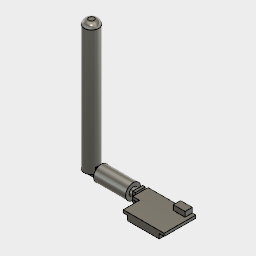
Video TX Module v1 (Autodesk Fusion 360 design; units mm, degrees)
Autodesk Fusion 360 part; units mm, degrees
note: some values were not read from the file. Set by a fixed rule: which sketch regions a step uses.
sketch "Sketch1" plane through (0, 0, 0) normal (0, 1, 0) x (1, 0, 0)
  line L0 (13.25, -10.25) -> (-13.25, -10.25)
  line L1 (-13.25, -10.25) -> (-13.25, 10.25)
  line L2 (-13.25, 10.25) -> (13.25, 10.25)
  line L3 (13.25, 10.25) -> (13.25, -10.25)
  line L4 (13.25, -10.25) -> (-13.25, 10.25) construction
  line L5 (-13.25, -10.25) -> (13.25, 10.25) construction
  line L6 (-13.25, 10.25) -> (-17.65, 10.25)
  line L7 (-17.65, 10.25) -> (-17.65, 0.25)
  line L8 (-17.65, 0.25) -> (-13.25, 0.25)
  dimension "d1" = 26.5
  dimension "d2" = 20.5
  dimension "d3" = 10
  dimension "d4" = 4.4
  measures "d1" distance of L1.end L2.end
  measures "d2" distance of L0.end L1.end
  measures "d3" distance of L6.end L7.end
  measures "d4" distance of L1.end L6.end
extrude "Extrude1" add sketch "Sketch1" along normal blind 1.85
sketch "Sketch2" plane through (0, 1.85, 0) normal (0, 1, 0) x (-1, 0, 0)
  line L0 (-13.25, -10.25) -> (17.65, -10.25)
  line L1 (17.65, -10.25) -> (17.65, -0.25)
  line L2 (17.65, -0.25) -> (13.25, -0.25)
  line L3 (13.25, -0.25) -> (13.25, 10.25)
  line L4 (13.25, 10.25) -> (-13.25, 10.25)
  line L5 (-13.25, 10.25) -> (-13.25, -10.25)
  line L6 (-11, -10.25) -> (-3.4, -10.25)
  line L7 (-3.4, -10.25) -> (-3.4, -5.55)
  line L8 (-3.4, -5.55) -> (-11, -5.55)
  line L9 (-11, -5.55) -> (-11, -10.25)
  dimension "d7" = 7.6
  dimension "d8" = 4.7
  dimension "d9" = 2.25
  measures "d7" distance of L6.start L6.end
  measures "d8" distance of L6.start L8.end
  measures "d9" distance of L5 L9
extrude "Extrude2" add sketch "Sketch2" along normal blind 3.2 contours L0 L6 L7 L8 L9
sketch "Sketch3" plane through (0, 0, 0) normal (0, -1, 0) x (1, 0, 0)
  line L0 (-17.65, -10.25) -> (13.25, -10.25)
  line L1 (13.25, -10.25) -> (13.25, 10.25)
  line L2 (13.25, 10.25) -> (-13.25, 10.25)
  line L3 (-13.25, 10.25) -> (-13.25, -0.25)
  line L4 (-13.25, -0.25) -> (-17.65, -0.25)
  line L5 (-17.65, -0.25) -> (-17.65, -10.25)
  line L6 (-10.5, 10.25) -> (10, 10.25)
  line L7 (10, 10.25) -> (10, -10.25)
  line L8 (10, -10.25) -> (-10.5, -10.25)
  line L9 (-10.5, -10.25) -> (-10.5, 10.25)
  dimension "d12" = 20.5
  dimension "d13" = 3.25
  measures "d12" distance of L7 L9
  measures "d13" distance of L1 L7
extrude "Extrude3" add sketch "Sketch3" along normal blind 3 contours L0 L2 L6 L7 L8 L9
sketch "Sketch4" plane through (-17.65, 0, 0) normal (-1, 0, 0) x (0, 0, 1)
  line L0 (-10.25, 0) -> (-0.25, 0)
  line L1 (-0.25, 0) -> (-0.25, 1.85)
  line L2 (-0.25, 1.85) -> (-10.25, 1.85)
  line L3 (-10.25, 1.85) -> (-10.25, 0)
  line L4 (-8.5, 3.05) -> (-2, 3.05)
  line L5 (-2, 3.05) -> (-2, -3.45)
  line L6 (-2, -3.45) -> (-8.5, -3.45)
  line L7 (-8.5, -3.45) -> (-8.5, 3.05)
  dimension "d16" = 6.5
  dimension "d17" = 6.5
  dimension "d18" = 1.2
  dimension "d19" = 1.75
  measures "d16" distance of L4.start L4.end
  measures "d17" distance of L4.start L6.end
  measures "d18" distance of L2 L4
  measures "d19" distance of L3 L7
extrude "Extrude4" add sketch "Sketch4" along normal blind 1.7 contours L0 L2 L5 L7 | L0 L5 L6 L7 | L2 L4 L5 L7
sketch "Sketch5" plane through (-19.35, 0, 0) normal (-1, 0, 0) x (0, 0, 1)
  line L0 (-8.5, -3.45) -> (-2, -3.45)
  line L1 (-2, -3.45) -> (-2, 3.05)
  line L2 (-2, 3.05) -> (-8.5, 3.05)
  line L3 (-8.5, 3.05) -> (-8.5, -3.45)
  circle A0 centre (-5.25, -0.2) radius 2.65
  line L4 (-5.25, -0.2) -> (-5.25, 3.05) construction
  line L5 (-5.25, -0.2) -> (-5.25, -3.45) construction
  dimension "d22" = 5.3
  measures "d22" diameter of A0
extrude "Extrude5" add sketch "Sketch5" along normal blind 2.85 contours A0
sketch "Sketch6" plane through (-22.2, 0, 0) normal (-1, 0, 0) x (0, 0, 1)
  circle A0 centre (-5.25, -0.2) radius 2.65
  circle A1 centre (-5.25, -0.2) radius 5
  dimension "d25" = 10
  measures "d25" diameter of A1
extrude "Extrude6" add sketch "Sketch6" along normal blind 20.75 contours A0 | A1
sketch "Sketch7" plane through (-42.95, 0, 0) normal (-1, 0, 0) x (0, 0, 1)
  circle A0 centre (-5.25, -0.2) radius 5
  line L0 (-3.5, -3.45) -> (-7, -3.45)
  line L1 (-7, -3.45) -> (-7, 3.05)
  line L2 (-7, 3.05) -> (-3.5, 3.05)
  line L3 (-3.5, 3.05) -> (-3.5, -3.45)
  line L4 (-3.5, -3.45) -> (-7, 3.05) construction
  line L5 (-7, -3.45) -> (-3.5, 3.05) construction
  point P0 (-5.25, -0.2)
  dimension "d28" = 6.5
  dimension "d29" = 3.5
  measures "d28" distance of L0.end L1.end
  measures "d29" distance of L1.end L2.end
extrude "Extrude7" add sketch "Sketch7" along normal blind 6.3 contours L0 L1 L2 L3
sketch "Sketch8" plane through (0, 3.05, 0) normal (0, 1, 0) x (-1, 0, 0)
  line L0 (42.95, -3.5) -> (42.95, -7)
  line L1 (42.95, -7) -> (49.25, -7)
  line L2 (49.25, -7) -> (49.25, -3.5)
  line L3 (49.25, -3.5) -> (42.95, -3.5)
  circle A0 centre (49.25, -5.25) radius 4.75
  dimension "d32" = 9.5
  measures "d32" diameter of A0
extrude "Extrude8" add sketch "Sketch8" along normal blind 80 contours L1 L2 L3 A0 | L1 L2 L3 A0
extrude "Extrude9" add 1 faces at (-50.8333, 3.05, -5.25) along direction (0, -1, 0) blind 4
fillet "Fillet1" radius 3 1 edges at (-44.8214, 83.05, -6.9677)
